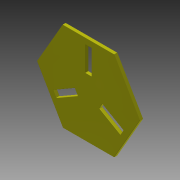
# Autodesk Inventor part: BASE002 - 300mm Plate
Saved by Autodesk Inventor 2015 SP1 (Build 190203100, 203)
## iProperties
Created: 2015-05-14
Part Number: BASE002 - 300mm Plate
Material: Generic
Document SubType Name: Modeling
Designer: rhornbak
Density: 1 g/cm^3
Appearance: Default
Author: rhornbak
Autodesk Inventor part; units mm, degrees
ref_plane "YZ Plane" through (0, 0, 0) normal (1, 0, 0) x (0, 1, 0)
ref_plane "XZ Plane" through (0, 0, 0) normal (0, 1, 0) x (-1, 0, 0)
ref_plane "XY Plane" through (0, 0, 0) normal (0, 0, 1) x (1, 0, 0)
sketch "Sketch1" plane through (0, 0, 0) normal (0, 1, 0) x (-1, 0, 0)
  line L0 (0, -173.2051) -> (150, 86.6025) construction
  line L1 (150, 86.6025) -> (-150, 86.6025) construction
  line L2 (-150, 86.6025) -> (0, -173.2051) construction
  line L3 (0, -169.0715) -> (0, 107.349) construction
  line L4 (10, 46.6025) -> (-10, 46.6025)
  line L5 (-10, 46.6025) -> (-10, 126.6025)
  line L6 (-10, 126.6025) -> (10, 126.6025)
  line L7 (10, 126.6025) -> (10, 46.6025)
  line L8 (-84.641, -146.6025) -> (-169.282, 0)
  line L9 (-84.641, 146.6025) -> (84.641, 146.6025)
  line L10 (169.282, 0) -> (84.641, -146.6025)
  line L11 (104.641, -71.9615) -> (35.359, -31.9615)
  line L12 (35.359, -31.9615) -> (45.359, -14.641)
  line L13 (45.359, -14.641) -> (114.641, -54.641)
  line L14 (114.641, -54.641) -> (104.641, -71.9615)
  line L15 (-35.359, -31.9615) -> (-104.641, -71.9615)
  line L16 (-104.641, -71.9615) -> (-114.641, -54.641)
  line L17 (-114.641, -54.641) -> (-45.359, -14.641)
  line L18 (-45.359, -14.641) -> (-35.359, -31.9615)
  line L19 (54.4642, -31.4449) -> (-94.6243, 54.6314) construction
  line L20 (94.7911, 54.7276) -> (-53.1844, -30.706) construction
  line L21 (-84.641, 146.6025) -> (-169.282, 0)
  line L22 (169.282, 0) -> (84.641, 146.6025)
  line L23 (84.641, -146.6025) -> (-84.641, -146.6025)
  point P0 (0, 0)
  dimension "SlotWidth" = 20
  dimension "SlotHeight" = 80
  dimension "SlotHeightCenterline" = 40
  dimension "d8" = 80
  dimension "d9" = 20
  dimension "d10" = 40
  dimension "EdgeThickness" = 20
  dimension "d12" = 20
  dimension "d13" = 80
  dimension "d14" = 20
  dimension "d15" = 40
  dimension "d16" = 20
  dimension "BaseCenterline" = 150
  dimension "d24" = 150
  dimension "PlateWidth" = 338.5641
  dimension "PlateHeight" = 293.2051
  constraints: 48 end point, 13 parallel, 5 equal length, 5 perpendicular, 3 point on line, 2 horizontal, 1 vertical, 4 other
  measures "SlotWidth" distance of L5.end L6.end
  measures "SlotHeight" distance of L4.end L5.end
  measures "SlotHeightCenterline" distance between parallel lines of L1 L4
  measures "d8" distance of L11.start L11.end
  measures "d9" distance of L13.end L11.start
  measures "d10" distance between parallel lines of L0 L12
  measures "EdgeThickness" distance between parallel lines of L9 L6
  measures "d12" distance between parallel lines of L10 L14
  measures "d13" distance of L15.start L15.end
  measures "d14" distance of L15.end L16.end
  measures "d15" distance between parallel lines of L2 L18
  measures "d16" distance between parallel lines of L8 L16
  measures "BaseCenterline" distance from line of L1.end L3
  measures "d24" distance from line of L19 L0.end
  measures "PlateWidth" distance of L8.end L10.start
  measures "PlateHeight" distance between parallel lines of L23 L9
extrude "Extrusion1" add sketch "Sketch1" along normal mid plane 10
fillet "Fillet1" radius 1 45 edges at (104.641, 0, -71.9615) (109.641, -5, -63.3013) (114.641, 0, -54.641) (109.641, 5, -63.3013) (80, -5, -34.641) (45.359, 0, -14.641) (80, 5, -34.641) (40.359, -5, -23.3013) (35.359, 0, -31.9615) (40.359, 5, -23.3013) (70, -5, -51.9615) (70, 5, -51.9615) (-35.359, 0, -31.9615) (-40.359, -5, -23.3013) (-45.359, 0, -14.641) (-40.359, 5, -23.3013) (-80, -5, -34.641) (-114.641, 0, -54.641) (-80, 5, -34.641) (-109.641, -5, -63.3013) (-104.641, 0, -71.9615) (-109.641, 5, -63.3013) (-70, -5, -51.9615) (-70, 5, -51.9615) (10, 0, 46.6025) (10, -5, 86.6025) (10, 0, 126.6025) (10, 5, 86.6025) (0, -5, 126.6025) (-10, 0, 126.6025) (0, 5, 126.6025) (-10, -5, 86.6025) (-10, 0, 46.6025) (-10, 5, 86.6025) (0, -5, 46.6025) (0, 5, 46.6025) (126.9615, -5, -73.3013) (0, -5, 146.6025) (-126.9615, -5, -73.3013) (169.282, 0, 0) (0, 5, 146.6025) (-84.641, 0, 146.6025) (-126.9615, 5, -73.3013) (-84.641, 0, -146.6025) (126.9615, 5, -73.3013)
equation "\"SlotHeightCenterline\" = 0.5 * SlotHeight"
equation "\"d8\" = SlotHeight"
equation "\"d9\" = SlotWidth"
equation "\"d10\" = SlotHeightCenterline"
equation "\"d12\" = EdgeThickness"
equation "\"d13\" = SlotHeight"
equation "\"d14\" = SlotWidth"
equation "\"d15\" = SlotHeightCenterline"
equation "\"d16\" = EdgeThickness"
equation "\"BaseCenterline\" = 0.5 * BaseLength"
equation "\"d24\" = BaseCenterline"
equation "\"BaseLength\" = 300"
body "Solid1"
